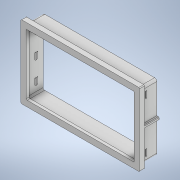
# Autodesk Inventor part: vw_mk4_double_din_adapter
Saved by Autodesk Inventor 2021 (Build 250183000, 183)
## iProperties
Created: 2022-05-31
Part Number: vw_mk4_double_din_adapter
Material: Generic
Document SubType Name: Modeling
Designer: Andrew
Density: 1 g/cm^3
Appearance: Default
Author: Andrew
Autodesk Inventor part; units mm, degrees
ref_plane "YZ Plane" through (0, 0, 0) normal (1, 0, 0) x (0, 1, 0)
ref_plane "XZ Plane" through (0, 0, 0) normal (0, 1, 0) x (-1, 0, 0)
ref_plane "XY Plane" through (0, 0, 0) normal (0, 0, 1) x (1, 0, 0)
sketch "Sketch1" plane through (0, 0, 0) normal (0, 0, 1) x (1, 0, 0)
  line L0 (-84.625, -48.65) -> (84.625, -48.65)
  line L1 (86.125, -47.15) -> (86.125, 47.15)
  line L2 (84.625, 48.65) -> (-84.625, 48.65)
  line L3 (-86.125, 47.15) -> (-86.125, -47.15)
  line L4 (-86.125, -48.65) -> (86.125, 48.65) construction
  line L5 (86.125, -48.65) -> (-86.125, 48.65) construction
  line L6 (-93.25, -58) -> (93.25, -58)
  line L7 (94.5, -56.75) -> (94.5, 56.75)
  line L8 (93.25, 58) -> (-93.25, 58)
  line L9 (-94.5, 56.75) -> (-94.5, -56.75)
  line L10 (-94.5, -58) -> (94.5, 58) construction
  line L11 (94.5, -58) -> (-94.5, 58) construction
  arc A0 (-84.625, 48.65) -> (-86.125, 47.15) centre (-84.625, 47.15) ccw
  arc A1 (84.625, -48.65) -> (86.125, -47.15) centre (84.625, -47.15) ccw
  arc A2 (86.125, 47.15) -> (84.625, 48.65) centre (84.625, 47.15) ccw
  arc A3 (-86.125, -47.15) -> (-84.625, -48.65) centre (-84.625, -47.15) ccw
  line L12 (-87.75, -52) -> (87.75, -52)
  line L13 (90.25, -49.5) -> (90.25, 49.5)
  line L14 (87.75, 52) -> (-87.75, 52)
  line L15 (-90.25, 49.5) -> (-90.25, -49.5)
  line L16 (-90.25, -52) -> (90.25, 52) construction
  line L17 (90.25, -52) -> (-90.25, 52) construction
  arc A4 (-93.25, 58) -> (-94.5, 56.75) centre (-93.25, 56.75) ccw
  arc A5 (-94.5, -56.75) -> (-93.25, -58) centre (-93.25, -56.75) ccw
  arc A6 (93.25, -58) -> (94.5, -56.75) centre (93.25, -56.75) ccw
  arc A7 (94.5, 56.75) -> (93.25, 58) centre (93.25, 56.75) ccw
  line L18 (90.25, -2.25) -> (94.5, -2.25)
  line L19 (94.5, -2.25) -> (94.5, 2.25)
  line L20 (94.5, 2.25) -> (90.25, 2.25)
  line L21 (90.25, 2.25) -> (90.25, -2.25)
  line L22 (90.25, -2.25) -> (94.5, 2.25) construction
  line L23 (94.5, -2.25) -> (90.25, 2.25) construction
  line L24 (87.5, -53) -> (-87.5, -53)
  line L25 (-91, -49.5) -> (-91, 49.5)
  line L26 (-87.5, 53) -> (87.5, 53)
  line L27 (91, 49.5) -> (91, -49.5)
  line L28 (91, -53) -> (-91, 53) construction
  line L29 (-91, -53) -> (91, 53) construction
  arc A8 (-87.75, 52) -> (-90.25, 49.5) centre (-87.75, 49.5) ccw
  arc A9 (-90.25, -49.5) -> (-87.75, -52) centre (-87.75, -49.5) ccw
  arc A10 (87.75, -52) -> (90.25, -49.5) centre (87.75, -49.5) ccw
  arc A11 (90.25, 49.5) -> (87.75, 52) centre (87.75, 49.5) ccw
  arc A12 (-87.5, 53) -> (-91, 49.5) centre (-87.5, 49.5) ccw
  arc A13 (-91, -49.5) -> (-87.5, -53) centre (-87.5, -49.5) ccw
  arc A14 (87.5, -53) -> (91, -49.5) centre (87.5, -49.5) ccw
  arc A15 (91, 49.5) -> (87.5, 53) centre (87.5, 49.5) ccw
  point P0 (0, 0)
  point P1 (92.375, 0)
  point P2 (92.375, 0)
  point P3 (0, 0)
  point P4 (90.25, 2.25)
  point P5 (90.25, -2.25)
  point P6 (94.5, -2.25)
  point P7 (91, 2.25)
  point P8 (91, -2.25)
  dimension "d0" = 189
  dimension "d1" = 116
  dimension "d2" = 172.25
  dimension "d3" = 97.3
  dimension "d6" = 1.5
  dimension "d7" = 180.5
  dimension "d8" = 104
  dimension "d9" = 1.25
  dimension "d12" = 4.5
  dimension "d64" = 182
  dimension "d66" = 1
  dimension "d70" = 2.5
  dimension "d71" = 3.5
  constraints: 60 end point, 33 point on line, 32 point on circle, 32 tangent, 16 centre point, 12 equal radius, 12 midpoint, 10 parallel, 5 horizontal, 5 perpendicular, 1 collinear, 1 horizontal alignment
  measures "d0" distance of L10.end L11.end
  measures "d1" distance of L11.start L10.end
  measures "d2" distance of L4.end L5.end
  measures "d3" distance of L5.start L4.end
  measures "d6" radius of A0
  measures "d7" distance of L16.end L17.end
  measures "d8" distance of L17.start L16.end
  measures "d9" radius of A4
  measures "d12" distance between parallel lines of L18 L20
  measures "d64" distance of L28.end L29.end
  measures "d66" distance between parallel lines of L14 L26
  measures "d70" radius of A8
  measures "d71" radius of A12
sketch "Sketch5" plane through (0, 0, 0) normal (0, 1, 0) x (-1, 0, 0)
  line L0 (-90.25, -22.5072) -> (-90.25, -18.0749)
  line L1 (-90.25, -18.0749) -> (-89.25, -18.7752)
  line L2 (-89.25, -18.7752) -> (-90.25, -22.5072)
  line L3 (-91, -15.0411) -> (-91, -12.8249)
  line L4 (-91, -12.8249) -> (-91.5, -13.1751)
  line L5 (-91.5, -13.1751) -> (-91, -15.0411)
  point P0 (0, 0)
  point P1 (-90.25, 0)
  point P2 (-90.25, 0)
  point P3 (-90.25, 0)
  point P4 (-90, -18.25)
  point P5 (-91.25, -13)
  point P6 (-91, 0)
  point P7 (-91, 0)
  point P8 (-91, 0)
  dimension "d75" = 15
  dimension "d85" = 1
  dimension "d87" = 55
  dimension "d88" = 0.25
  dimension "d89" = 18.25
  dimension "d90" = 15
  dimension "d91" = 55
  dimension "d92" = 0.25
  dimension "d93" = 13
  dimension "d94" = 0.5
  constraints: 12 end point, 3 point on line, 2 vertical, 1 midpoint
  measures "d75" angle of L2 L0
  measures "d85" distance from line of L0 L1.end
  measures "d87" angle of L0 L1
  measures "d88" distance from line of L0 point (-90, -18.25)
  measures "d89" vertical distance of point (-90.25, 0) point (-90, -18.25)
  measures "d90" angle of L3 L5
  measures "d91" angle of L3 L4
  measures "d92" distance from line of L3 point (-91.25, -13)
  measures "d93" vertical distance of point (0, 0) point (-91.25, -13)
  measures "d94" distance from line of L4.end L3
extrude "Extrusion1" add sketch "Sketch1" against normal blind 4.5
extrude "Extrusion8" add sketch "Sketch1" against normal blind 7.75 contours A5 L9 A4 L8 A7 L7 L20 L27 A15 L26 A12 L25 A13 L24 A14 L18 A6 L6
extrude "Extrusion2" add sketch "Sketch1" against normal blind 31 contours L18 L27 L20 L7 | L18 L13 L20 L27
fillet "Fillet3" radius 1 2 edges at (94.5, 2.25, -19.375) (94.5, -2.25, -19.375)
mirror "Mirror1" about plane through (0, 0, 0) normal (1, 0, 0) of "Extrusion2", "Fillet3"
extrude "Extrusion3" add sketch "Sketch1" against normal blind 31 contours L27 A14 L24 A13 L25 A12 L26 A15 L20 L13 A11 L14 A8 L15 A9 L12 A10 L18 | L18 L13 L20 L27
extrude "Extrusion9" add sketch "Sketch5" along normal blind 40 separate body contours L0 L1 L2
extrude "Extrusion10" cut sketch "Sketch5" along normal blind 30 contours L0 L1 L2 bodies 2
extrude "Extrusion11" add sketch "Sketch5" along normal blind 5 contours L0 L1 L2 bodies 2
mirror "Mirror4" about plane through (0, 0, 0) normal (0, 1, 0) bodies 2
mirror "Mirror5" about plane through (0, 0, 0) normal (1, 0, 0) bodies 2
combine bodies "Combine2" operation type add bodies to combine 1 2
extrude "Extrusion12" add sketch "Sketch5" along normal blind 45 separate body contours L5 L4 L3
extrude "Extrusion13" cut sketch "Sketch5" along normal blind 35 contours L5 L4 L3 bodies 3
mirror "Mirror6" about plane through (0, 0, 0) normal (0, 1, 0) bodies 3
mirror "Mirror7" about plane through (0, 0, 0) normal (1, 0, 0) bodies 3
combine bodies "Combine3" operation type add bodies to combine 1 3
equation "\"d15\" = d13"
equation "\"mount_width\" = 166.5"
equation "\"d13\" = 31"
body "Solid1"
